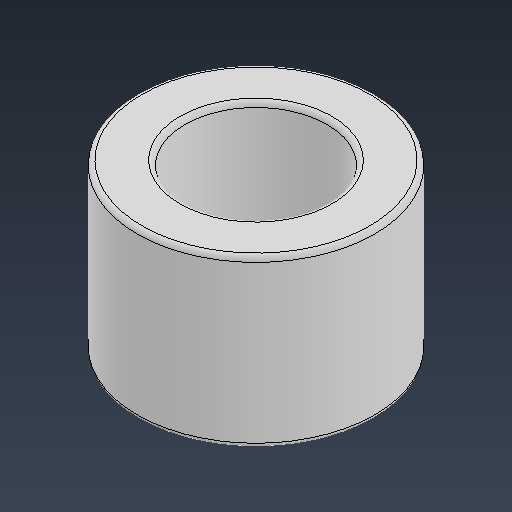
# Autodesk Inventor part: ball-bearing
Saved by Autodesk Inventor 2026.2 (Build 302298010, 298A)
## iProperties
Created: 2025-06-29
Part Number: ball-bearing
Material: Generic
Document SubType Name: Modeling
Designer: szymo
Density: 4.55846 g/cm^3
Appearance: Default
Mass: 1.6 g
Surface Area: 4.4376 cm^2
Volume: 0.350995 cm^3
Author: szymo
Autodesk Inventor part; units mm, degrees
ref_plane "YZ Plane" through (0, 0, 0) normal (1, 0, 0) x (0, 1, 0)
ref_plane "XZ Plane" through (0, 0, 0) normal (0, 1, 0) x (-1, 0, 0)
ref_plane "XY Plane" through (0, 0, 0) normal (0, 0, 1) x (1, 0, 0)
sketch "Sketch1" plane through (0, 0, 0) normal (0, 1, 0) x (-1, 0, 0)
  circle A0 centre (0, 0) radius 3
  circle A1 centre (0, 0) radius 5
  dimension "d0" = 6
  dimension "d1" = 10
  constraints: 2 centre point, 2 coincident
  measures "d0" diameter of A0
  measures "d1" diameter of A1
extrude "Extrusion1" add sketch "Sketch1" along normal blind 7
fillet "Fillet1" radius 0.2 4 edges at (3, 7, 0) (5, 7, 0) (3, 0, 0) (5, 0, 0)
body "Solid1"
